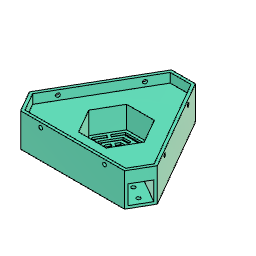
lower_connector (Autodesk Fusion 360 design; units mm, degrees)
Autodesk Fusion 360 part; units mm, degrees
sketch "Sketch1" plane through (0, 0, 0) normal (0, 0, 1) x (1, 0, 0)
  line L0 (-26, 0) -> (-82.282, -97.4833)
  line L1 (-69.282, -120) -> (43.282, -120)
  line L2 (56.282, -97.4833) -> (0, 0)
  line L3 (49.782, -108.7417) -> (-54.141, -48.7417) construction
  line L4 (0, 0) -> (-26, 0)
  line L5 (-82.282, -97.4833) -> (-69.282, -120)
  line L6 (43.282, -120) -> (56.282, -97.4833)
  line L7 (-13, 0) -> (-13, -120) construction
  line L8 (-75.782, -108.7417) -> (28.141, -48.7417) construction
  line L9 (-24.2679, -3) -> (-78.8179, -97.4833)
  line L10 (-78.8179, -97.4833) -> (-67.55, -117)
  line L11 (-67.55, -117) -> (41.55, -117)
  line L12 (41.55, -117) -> (52.8179, -97.4833)
  line L13 (52.8179, -97.4833) -> (-1.7321, -3)
  line L14 (-1.7321, -3) -> (-24.2679, -3)
  line L15 (2, -98.4752) -> (-28, -98.4752)
  line L16 (-28, -98.4752) -> (-43, -72.4944)
  line L17 (-43, -72.4944) -> (-28, -46.5137)
  line L18 (-28, -46.5137) -> (2, -46.5137)
  line L19 (2, -46.5137) -> (17, -72.4944)
  line L20 (17, -72.4944) -> (2, -98.4752)
  point P0 (-13, -72.4944)
  dimension "d18" = 120
  dimension "d25" = -3
  dimension "d36" = 26
  dimension "d42" = 30
  constraint coincident L2.end L4.start
  constraint horizontal L1
  constraint midpoint L0 L3.end
  constraint coincident L3 P0
  constraint symmetric L1.end L2.start L3
  constraint coincident L3.start L6
  constraint horizontal L4
  constraint midpoint L4 L7.start
  constraint midpoint L1 L7.end
  constraint midpoint L5 L8.start
  constraint midpoint L2 L8.end
  constraint coincident P0 L8
  constraint coincident P0 L7
  constraint perpendicular L4 L7
  constraint perpendicular L5 L8
  constraint symmetric L0 L1 L8
  constraint symmetric L0 L2 L7
  constraint equal L1 L2
  constraint horizontal L15
  constraint perpendicular L8 L16
  constraint parallel L15 L18
  constraint perpendicular L3 L20
  constraint perpendicular L8 L19
  constraint perpendicular L3 L17
  constraint symmetric L7 L16 L20
  constraint symmetric L7 L17 L19
  constraint symmetric L3 L16 L18
  constraint symmetric L3 L15 L19
  constraint equal L15 L16
  measures "d18" distance of L2.end L1
  measures "d36" distance of L1.end L2.start
  measures "d42" distance of L15.start L15.end
extrude "Extrude7" add sketch "Sketch1" along normal blind 2 contours L15 L16 L17 L18 L19 L20
extrude "Extrude4" add sketch "Sketch1" along normal blind 26 contours L0 L1 L2 L4 L5 L6 | L9 L10 L11 L12 L13 L14
sketch "Sketch2" plane through (84.423, -48.7417, 0) normal (0.866025, -0.5, 0) x (0.5, 0.866025, 0)
  line L0 (-82.282, 0) -> (-56.282, 0)
  line L1 (-56.282, 0) -> (-56.282, 26)
  line L2 (-56.282, 26) -> (-82.282, 26)
  line L3 (-82.282, 26) -> (-82.282, 0)
  line L4 (-82.282, 0) -> (-56.282, 26) construction
  line L5 (-56.282, 0) -> (-82.282, 26) construction
  line L6 (-79.482, 2.8) -> (-59.082, 2.8)
  line L7 (-59.082, 2.8) -> (-59.082, 23.2)
  line L8 (-59.082, 23.2) -> (-79.482, 23.2)
  line L9 (-79.482, 23.2) -> (-79.482, 2.8)
  dimension "d79" = 20.4
  constraint coincident L0.start L3.end
  constraint coincident L1.end L2.start
  constraint coincident L0.end L1.start
  constraint coincident L2.end L3.start
  constraint horizontal L6
  constraint vertical L7
  constraint horizontal L8
  constraint vertical L9
  constraint coincident L4 L7.end
  constraint coincident L4 L6.start
  constraint coincident L5 L8.end
  measures "d79" distance of L7.end L8.end
extrude "Extrude5" cut sketch "Sketch2" against normal blind 30 contours L6 L7 L8 L9
sketch "Sketch8" plane through (0, 0, 0) normal (0, 1, 0) x (-1, 0, 0)
  line L0 (0, 0) -> (26, 0)
  line L1 (26, 0) -> (26, 26)
  line L2 (26, 26) -> (0, 26)
  line L3 (0, 26) -> (0, 0)
  line L4 (0, 0) -> (26, 26) construction
  line L5 (0, 26) -> (26, 0) construction
  line L6 (2.8, 2.8) -> (23.2, 2.8)
  line L7 (23.2, 2.8) -> (23.2, 23.2)
  line L8 (23.2, 23.2) -> (2.8, 23.2)
  line L9 (2.8, 23.2) -> (2.8, 2.8)
  dimension "d62" = 20.4
  constraint coincident L0.start L3.end
  constraint coincident L1.end L2.start
  constraint coincident L2.end L3.start
  constraint coincident L0.end L1.start
  constraint horizontal L6
  constraint vertical L7
  constraint horizontal L8
  constraint vertical L9
  constraint coincident L4 L7.end
  constraint coincident L4 L6.start
  constraint coincident L5 L8.end
  measures "d62" distance of L7.end L8.end
extrude "Extrude9" cut sketch "Sketch8" against normal blind 30 contours L6 L7 L8 L9
sketch "Sketch9" plane through (-103.923, -60, 0) normal (-0.866025, -0.5, 0) x (0.5, -0.866025, 0)
  line L0 (43.282, 0) -> (69.282, 0)
  line L1 (69.282, 0) -> (69.282, 26)
  line L2 (69.282, 26) -> (43.282, 26)
  line L3 (43.282, 26) -> (43.282, 0)
  line L4 (43.282, 0) -> (69.282, 26) construction
  line L5 (43.282, 26) -> (69.282, 0) construction
  line L6 (46.082, 2.8) -> (66.482, 2.8)
  line L7 (66.482, 2.8) -> (66.482, 23.2)
  line L8 (66.482, 23.2) -> (46.082, 23.2)
  line L9 (46.082, 23.2) -> (46.082, 2.8)
  dimension "d65" = 20.4
  constraint coincident L0.start L3.end
  constraint coincident L1.end L2.start
  constraint coincident L2.end L3.start
  constraint coincident L0.end L1.start
  constraint horizontal L6
  constraint vertical L7
  constraint horizontal L8
  constraint vertical L9
  constraint coincident L4 L7.end
  constraint coincident L4 L6.start
  constraint coincident L5 L8.end
  measures "d65" distance of L7.end L8.end
extrude "Extrude10" cut sketch "Sketch9" against normal blind 30 contours L6 L7 L8 L9
sketch "Sketch7" plane through (0, 0, 2) normal (0, 0, 1) x (-1, 0, 0)
  line L0 (14.5, 80.4752, 24) -> (14.5, 83.4752, 24)
  line L1 (17.6077, 80.4752, 24) -> (14.5, 80.4752, 24)
  line L2 (24.3577, 80.7839, 24) -> (26.9558, 82.2839, 24)
  line L3 (18.7513, 72.4944, 24) -> (18.0635, 73.6858, 24)
  line L4 (25.6795, 72.4944, 24) -> (19.3397, 83.4752, 24)
  line L5 (22.2154, 72.4944, 24) -> (20.6615, 75.1858, 24)
  line L6 (19.1615, 77.7839, 24) -> (17.6077, 80.4752, 24)
  line L7 (24.3577, 80.7839, 24) -> (21.0718, 86.4752, 24)
  line L8 (20.6615, 75.1858, 24) -> (19.1615, 77.7839, 24)
  line L9 (19.3397, 83.4752, 24) -> (14.5, 83.4752, 24)
  line L10 (18.0635, 73.6858, 24) -> (20.6615, 75.1858, 24)
  line L11 (25.8577, 78.1858, 24) -> (28.4558, 79.6858, 24)
  line L12 (16.5635, 76.2839, 24) -> (15.8756, 77.4752, 24)
  line L13 (18.0635, 73.6858, 24) -> (16.5635, 76.2839, 24)
  line L14 (15.8756, 77.4752, 24) -> (10.1244, 77.4752, 24)
  line L15 (16.5635, 76.2839, 24) -> (19.1615, 77.7839, 24)
  line L16 (26.2679, 95.4752, 24) -> (14.5, 95.4752, 24)
  line L17 (24.5359, 92.4752, 24) -> (14.5, 92.4752, 24)
  line L18 (29.1436, 72.4944, 24) -> (25.8577, 78.1858, 24)
  line L19 (6.6603, 61.5137, 24) -> (19.3397, 61.5137, 24)
  line L20 (26.9558, 82.2839, 24) -> (22.8038, 89.4752, 24)
  line L21 (14.5, 58.5137, 24) -> (21.0718, 58.5137, 24)
  line L22 (14.5, 55.5137, 24) -> (22.8038, 55.5137, 24)
  line L23 (11.5, 64.5137, 24) -> (14.5, 64.5137, 24)
  line L24 (14.5, 92.4752, 24) -> (14.5, 95.4752, 24)
  line L25 (19.3397, 61.5137, 24) -> (21.7596, 65.705, 24)
  line L26 (17.6077, 64.5137, 24) -> (19.1615, 67.205, 24)
  line L27 (32.6077, 72.4944, 24) -> (28.4558, 79.6858, 24)
  line L28 (34.75, 58.205, 24) -> (-10.25, 84.1858, 24) construction
  line L29 (4.2404, 65.705, 24) -> (2.7404, 68.3031, 24)
  line L30 (3.1962, 55.5137, 24) -> (11.5, 55.5137, 24)
  line L31 (10.1244, 67.5137, 24) -> (11.5, 67.5137, 24)
  line L32 (5.3385, 69.8031, 24) -> (2.7404, 68.3031, 24)
  line L33 (3.7846, 72.4944, 24) -> (5.3385, 69.8031, 24)
  line L34 (7.2487, 72.4944, 24) -> (10.1244, 67.5137, 24)
  line L35 (-0.2679, 49.5137, 24) -> (26.2679, 49.5137, 24)
  line L36 (0.3205, 72.4944, 24) -> (2.7404, 68.3031, 24)
  line L37 (6.8385, 67.205, 24) -> (5.3385, 69.8031, 24)
  line L38 (-13.5359, 72.4944, 24) -> (-7.6519, 62.3031, 24)
  line L39 (-2, 46.5137, 24) -> (28, 46.5137, 24)
  line L40 (-2, 98.4752, 24) -> (-17, 72.4944, 24)
  line L41 (11.5, 98.4752, 24) -> (11.5, 46.5137, 24) construction
  line L42 (-6.6077, 72.4944, 24) -> (3.1962, 55.5137, 24)
  line L43 (-17, 72.4944, 24) -> (-2, 46.5137, 24)
  line L44 (11.5, 67.5137, 24) -> (11.5, 64.5137, 24)
  line L45 (8.3923, 64.5137, 24) -> (11.5, 64.5137, 24)
  line L46 (34.75, 86.7839, 24) -> (-10.25, 60.8031, 24) construction
  line L47 (11.5, 58.5137, 24) -> (11.5, 55.5137, 24)
  line L48 (4.2404, 65.705, 24) -> (6.6603, 61.5137, 24)
  line L49 (6.8385, 67.205, 24) -> (4.2404, 65.705, 24)
  line L50 (6.8385, 67.205, 24) -> (8.3923, 64.5137, 24)
  line L51 (-3.5538, 61.205, 24) -> (1.4641, 52.5137, 24)
  line L52 (-9.5, 59.5041, 24) -> (35.5, 85.4848, 24) construction
  line L53 (4.9282, 58.5137, 24) -> (11.5, 58.5137, 24)
  line L54 (-10.0718, 72.4944, 24) -> (-5.0538, 63.8031, 24)
  line L55 (36.25, 84.1858, 24) -> (-8.75, 58.205, 24) construction
  line L56 (23.2596, 68.3031, 24) -> (25.6795, 72.4944, 24)
  line L57 (15.8756, 67.5137, 24) -> (18.7513, 72.4944, 24)
  line L58 (26.2679, 49.5137, 24) -> (32.1519, 59.705, 24)
  line L59 (31.0538, 63.8031, 24) -> (36.0718, 72.4944, 24)
  line L60 (22.8038, 55.5137, 24) -> (32.6077, 72.4944, 24)
  line L61 (19.1615, 67.205, 24) -> (21.7596, 65.705, 24)
  line L62 (36.0718, 72.4944, 24) -> (24.5359, 92.4752, 24)
  line L63 (14.5, 64.5137, 24) -> (17.6077, 64.5137, 24)
  line L64 (43, 72.4944, 24) -> (28, 98.4752, 24)
  line L65 (39.5359, 72.4944, 24) -> (26.2679, 95.4752, 24)
  line L66 (29.5538, 61.205, 24) -> (32.1519, 59.705, 24)
  line L67 (19.1615, 67.205, 24) -> (20.6615, 69.8031, 24)
  line L68 (21.7596, 65.705, 24) -> (23.2596, 68.3031, 24)
  line L69 (28, 46.5137, 24) -> (43, 72.4944, 24)
  line L70 (14.5, 67.5137, 24) -> (15.8756, 67.5137, 24)
  line L71 (11.5, 67.5137, 24) -> (14.5, 67.5137, 24)
  line L72 (14.5, 64.5137, 24) -> (14.5, 67.5137, 24)
  line L73 (23.2596, 68.3031, 24) -> (20.6615, 69.8031, 24)
  line L74 (14.5, 55.5137, 24) -> (14.5, 58.5137, 24)
  line L75 (14.5, 46.5137, 24) -> (14.5, 98.4752, 24) construction
  line L76 (21.0718, 58.5137, 24) -> (29.1436, 72.4944, 24)
  line L77 (24.5359, 52.5137, 24) -> (29.5538, 61.205, 24)
  line L78 (20.6615, 69.8031, 24) -> (22.2154, 72.4944, 24)
  line L79 (5.3385, 75.1858, 24) -> (6.8385, 77.7839, 24)
  line L80 (13, 98.4752, 24) -> (13, 46.5137, 24) construction
  line L81 (33.6519, 62.3031, 24) -> (39.5359, 72.4944, 24)
  line L82 (33.6519, 62.3031, 24) -> (31.0538, 63.8031, 24)
  line L83 (1.4641, 52.5137, 24) -> (24.5359, 52.5137, 24)
  line L84 (-3.1436, 72.4944, 24) -> (4.9282, 58.5137, 24)
  line L85 (36.25, 60.8031, 24) -> (-8.75, 86.7839, 24) construction
  line L86 (35.5, 59.5041, 24) -> (-9.5, 85.4848, 24) construction
  line L87 (1.4641, 92.4752, 24) -> (-10.0718, 72.4944, 24)
  line L88 (-0.2679, 95.4752, 24) -> (-13.5359, 72.4944, 24)
  line L89 (-3.5538, 61.205, 24) -> (-6.1519, 59.705, 24)
  line L90 (22.8038, 89.4752, 24) -> (3.1962, 89.4752, 24)
  line L91 (11.5, 83.4752, 24) -> (6.6603, 83.4752, 24)
  line L92 (8.3923, 80.4752, 24) -> (6.8385, 77.7839, 24)
  line L93 (5.3385, 75.1858, 24) -> (3.7846, 72.4944, 24)
  line L94 (28, 98.4752, 24) -> (-2, 98.4752, 24)
  line L95 (3.1962, 89.4752, 24) -> (-0.9558, 82.2839, 24)
  line L96 (11.5, 92.4752, 24) -> (1.4641, 92.4752, 24)
  line L97 (-5.0538, 63.8031, 24) -> (-7.6519, 62.3031, 24)
  line L98 (11.5, 83.4752, 24) -> (11.5, 80.4752, 24)
  line L99 (21.0718, 86.4752, 24) -> (4.9282, 86.4752, 24)
  line L100 (-6.1519, 59.705, 24) -> (-0.2679, 49.5137, 24)
  line L101 (4.9282, 86.4752, 24) -> (1.6423, 80.7839, 24)
  line L102 (-2.4558, 79.6858, 24) -> (-6.6077, 72.4944, 24)
  line L103 (-2.4558, 79.6858, 24) -> (0.1423, 78.1858, 24)
  line L104 (11.5, 95.4752, 24) -> (-0.2679, 95.4752, 24)
  line L105 (2.7404, 76.6858, 24) -> (0.3205, 72.4944, 24)
  line L106 (4.2404, 79.2839, 24) -> (2.7404, 76.6858, 24)
  line L107 (7.9365, 73.6858, 24) -> (7.2487, 72.4944, 24)
  line L108 (11.5, 95.4752, 24) -> (11.5, 92.4752, 24)
  line L109 (10.1244, 77.4752, 24) -> (9.4365, 76.2839, 24)
  line L110 (1.6423, 80.7839, 24) -> (-0.9558, 82.2839, 24)
  line L111 (11.5, 80.4752, 24) -> (8.3923, 80.4752, 24)
  line L112 (9.4365, 76.2839, 24) -> (6.8385, 77.7839, 24)
  line L113 (7.9365, 73.6858, 24) -> (5.3385, 75.1858, 24)
  line L114 (7.9365, 73.6858, 24) -> (9.4365, 76.2839, 24)
  line L115 (0.1423, 78.1858, 24) -> (-3.1436, 72.4944, 24)
  line L116 (6.6603, 83.4752, 24) -> (4.2404, 79.2839, 24)
  dimension "d80" = 3
  dimension "d81" = 3
  dimension "d82" = 3
  dimension "d83" = 3
  dimension "d84" = 3
  dimension "d85" = 3
  dimension "d86" = 6
  dimension "d87" = 6
  dimension "d88" = 6
  dimension "d89" = 6
  dimension "d90" = 6
  dimension "d91" = 6
  dimension "d92" = 9
  dimension "d93" = 9
  dimension "d94" = 9
  dimension "d95" = 9
  dimension "d96" = 9
  dimension "d97" = 9
  dimension "d98" = 12
  dimension "d99" = 12
  dimension "d100" = 12
  dimension "d101" = 12
  dimension "d102" = 12
  dimension "d103" = 12
  dimension "d104" = 18
  dimension "d105" = 18
  dimension "d106" = 18
  dimension "d107" = 18
  dimension "d108" = 18
  dimension "d109" = 18
  dimension "d110" = 15
  dimension "d111" = 15
  dimension "d112" = 15
  dimension "d113" = 15
  dimension "d114" = 15
  dimension "d115" = 15
  dimension "d116" = 3
  dimension "d117" = 3
  dimension "d118" = 3
  dimension "d119" = 21
  dimension "d120" = 21
  dimension "d121" = 21
  dimension "d122" = 21
  dimension "d123" = 21
  dimension "d124" = 21
extrude "Extrude8" cut sketch "Sketch7" against normal blind 65 contours L0 L1 L4 L5 L6 L8 L9 L56 L73 L78 | L3 L12 L13 L14 L31 L34 L57 L70 L71 L107 L109 L114 | L19 L23 L25 L26 L45 L48 L49 L50 L61 L63 | L32 L33 L36 L79 L91 L92 L93 L98 L105 L106 L111 L116 | L2 L7 L20 L90 L95 L99 L101 L110 | L11 L18 L21 L22 L27 L60 L74 L76 | L16 L17 L24 L59 L62 L65 L81 L82 | L30 L42 L47 L53 L84 L102 L103 L115 | L35 L51 L58 L66 L77 L83 L89 L100 | L38 L54 L87 L88 L96 L97 L104 L108 in plane through (0, 0, 26) normal (0, 0, 1)
sketch "Sketch13" plane through (0, 0, 0) normal (0, 0, -1) x (1, 0, 0)
  line L0 (-6.6603, 83.4752) -> (-0.3205, 72.4944)
  line L1 (-0.3205, 72.4944) -> (-2.7404, 68.3031)
  line L2 (-2.7404, 68.3031) -> (-5.3385, 69.8031)
  line L3 (-5.3385, 69.8031) -> (-3.7846, 72.4944)
  line L4 (-3.7846, 72.4944) -> (-8.3923, 80.4752)
  line L5 (-8.3923, 80.4752) -> (-11.5, 80.4752)
  line L6 (-11.5, 80.4752) -> (-11.5, 83.4752)
  line L7 (-11.5, 83.4752) -> (-6.6603, 83.4752)
  line L8 (6.6077, 72.4944) -> (-3.1962, 55.5137)
  line L9 (-3.1962, 55.5137) -> (-11.5, 55.5137)
  line L10 (-11.5, 55.5137) -> (-11.5, 58.5137)
  line L11 (-11.5, 58.5137) -> (-4.9282, 58.5137)
  line L12 (-4.9282, 58.5137) -> (3.1436, 72.4944)
  line L13 (3.1436, 72.4944) -> (-0.1423, 78.1858)
  line L14 (-0.1423, 78.1858) -> (2.4558, 79.6858)
  line L15 (2.4558, 79.6858) -> (6.6077, 72.4944)
  line L16 (-26.2679, 95.4752) -> (-14.5, 95.4752)
  line L17 (-14.5, 95.4752) -> (-14.5, 92.4752)
  line L18 (-14.5, 92.4752) -> (-24.5359, 92.4752)
  line L19 (-24.5359, 92.4752) -> (-36.0718, 72.4944)
  line L20 (-36.0718, 72.4944) -> (-31.0538, 63.8031)
  line L21 (-31.0538, 63.8031) -> (-33.6519, 62.3031)
  line L22 (-33.6519, 62.3031) -> (-39.5359, 72.4944)
  line L23 (-39.5359, 72.4944) -> (-26.2679, 95.4752)
  line L24 (6.1519, 59.705) -> (0.2679, 49.5137)
  line L25 (0.2679, 49.5137) -> (-26.2679, 49.5137)
  line L26 (-26.2679, 49.5137) -> (-32.1519, 59.705)
  line L27 (-32.1519, 59.705) -> (-29.5538, 61.205)
  line L28 (-29.5538, 61.205) -> (-24.5359, 52.5137)
  line L29 (-24.5359, 52.5137) -> (-1.4641, 52.5137)
  line L30 (-1.4641, 52.5137) -> (3.5538, 61.205)
  line L31 (3.5538, 61.205) -> (6.1519, 59.705)
  line L32 (-4.2404, 65.705) -> (-6.6603, 61.5137)
  line L33 (-6.6603, 61.5137) -> (-19.3397, 61.5137)
  line L34 (-19.3397, 61.5137) -> (-21.7596, 65.705)
  line L35 (-21.7596, 65.705) -> (-19.1615, 67.205)
  line L36 (-19.1615, 67.205) -> (-17.6077, 64.5137)
  line L37 (-17.6077, 64.5137) -> (-8.3923, 64.5137)
  line L38 (-8.3923, 64.5137) -> (-6.8385, 67.205)
  line L39 (-6.8385, 67.205) -> (-4.2404, 65.705)
  line L40 (-25.6795, 72.4944) -> (-19.3397, 83.4752)
  line L41 (-19.3397, 83.4752) -> (-14.5, 83.4752)
  line L42 (-14.5, 83.4752) -> (-14.5, 80.4752)
  line L43 (-14.5, 80.4752) -> (-17.6077, 80.4752)
  line L44 (-17.6077, 80.4752) -> (-22.2154, 72.4944)
  line L45 (-22.2154, 72.4944) -> (-20.6615, 69.8031)
  line L46 (-20.6615, 69.8031) -> (-23.2596, 68.3031)
  line L47 (-23.2596, 68.3031) -> (-25.6795, 72.4944)
  line L48 (-26.9558, 82.2839) -> (-22.8038, 89.4752)
  line L49 (-22.8038, 89.4752) -> (-3.1962, 89.4752)
  line L50 (-3.1962, 89.4752) -> (0.9558, 82.2839)
  line L51 (0.9558, 82.2839) -> (-1.6423, 80.7839)
  line L52 (-1.6423, 80.7839) -> (-4.9282, 86.4752)
  line L53 (-4.9282, 86.4752) -> (-21.0718, 86.4752)
  line L54 (-21.0718, 86.4752) -> (-24.3577, 80.7839)
  line L55 (-24.3577, 80.7839) -> (-26.9558, 82.2839)
  line L56 (13.5359, 72.4944) -> (7.6519, 62.3031)
  line L57 (7.6519, 62.3031) -> (5.0538, 63.8031)
  line L58 (5.0538, 63.8031) -> (10.0718, 72.4944)
  line L59 (10.0718, 72.4944) -> (-1.4641, 92.4752)
  line L60 (-1.4641, 92.4752) -> (-11.5, 92.4752)
  line L61 (-11.5, 92.4752) -> (-11.5, 95.4752)
  line L62 (-11.5, 95.4752) -> (0.2679, 95.4752)
  line L63 (0.2679, 95.4752) -> (13.5359, 72.4944)
  line L64 (-22.8038, 55.5137) -> (-32.6077, 72.4944)
  line L65 (-32.6077, 72.4944) -> (-28.4558, 79.6858)
  line L66 (-28.4558, 79.6858) -> (-25.8577, 78.1858)
  line L67 (-25.8577, 78.1858) -> (-29.1436, 72.4944)
  line L68 (-29.1436, 72.4944) -> (-21.0718, 58.5137)
  line L69 (-21.0718, 58.5137) -> (-14.5, 58.5137)
  line L70 (-14.5, 58.5137) -> (-14.5, 55.5137)
  line L71 (-14.5, 55.5137) -> (-22.8038, 55.5137)
  line L72 (-10.1244, 67.5137) -> (-15.8756, 67.5137)
  line L73 (-15.8756, 67.5137) -> (-18.7513, 72.4944)
  line L74 (-18.7513, 72.4944) -> (-15.8756, 77.4752)
  line L75 (-15.8756, 77.4752) -> (-10.1244, 77.4752)
  line L76 (-10.1244, 77.4752) -> (-7.2487, 72.4944)
  line L77 (-7.2487, 72.4944) -> (-10.1244, 67.5137)
  line L78 (56.282, 97.4833) -> (43.282, 120)
  line L79 (43.282, 120) -> (-69.282, 120)
  line L80 (-69.282, 120) -> (-82.282, 97.4833)
  line L81 (-82.282, 97.4833) -> (-26, 0)
  line L82 (-26, 0) -> (0, 0)
  line L83 (0, 0) -> (56.282, 97.4833)
  line L84 (-13, 0) -> (-13, 72.4944) construction
  line L85 (-13, 72.4944) -> (49.782, 108.7417) construction
  line L86 (-13, 72.4944) -> (-75.782, 108.7417) construction
  circle A0 centre (-13, 7.5) radius 2
  circle A1 centre (-13, 22.5) radius 2
  circle A2 centre (43.2868, 104.9917) radius 2
  circle A3 centre (30.2965, 97.4917) radius 2
  circle A4 centre (-69.2868, 104.9917) radius 2
  circle A5 centre (-56.2965, 97.4917) radius 2
  dimension "d136" = 4
  dimension "d137" = 7.5
  dimension "d138" = 15
  dimension "d139" = 7.5
  dimension "d140" = 15
  dimension "d141" = 7.5
  dimension "d142" = 15
  constraint midpoint L82 L84.start
  constraint perpendicular L82 L84
  constraint midpoint L78 L85.end
  constraint midpoint L80 L86.end
  constraint perpendicular L80 L86
  constraint coincident L84 A0.centre
  constraint coincident L84 A1.centre
  constraint coincident L85 A2.centre
  constraint coincident L85 A3.centre
  constraint coincident L86 A4.centre
  constraint coincident L86 A5.centre
  constraint equal A0 A1
  constraint equal A1 A5
  constraint equal A4 A5
  constraint equal A3 A4
  constraint equal A2 A3
  measures "d136" diameter of A2
  measures "d137" distance of L78 A2.centre
  measures "d138" distance of A2.centre A3.centre
  measures "d139" distance of L82 A0.centre
  measures "d140" distance of A0.centre A1.centre
  measures "d141" distance of L80 A4.centre
  measures "d142" distance of A4.centre A5.centre
extrude "Extrude14" cut sketch "Sketch13" against normal blind 10 contours A0 | A1 | A2 | A3 | A4 | A5
extrude "Extrude16" add sketch "Sketch1" along normal blind 10 from surface at 26 contours L0 L1 L2 L4 L5 L6
sketch "Sketch17" plane through (-16.9019, 9.7583, 0) normal (0.866025, -0.5, 0) x (0.5, 0.866025, 0)
  line L0 (-123.832, 26) -> (-14.7321, 26)
  line L1 (-14.7321, 26) -> (-14.7321, 36)
  line L2 (-14.7321, 36) -> (-123.832, 36)
  line L3 (-123.832, 36) -> (-123.832, 26)
  line L4 (-123.832, 31) -> (-14.7321, 31) construction
  line L5 (-69.282, 26) -> (-69.282, 36) construction
  circle A0 centre (-103.832, 31) radius 2
  circle A1 centre (-34.7321, 31) radius 2
  dimension "d154" = 20
  dimension "d155" = 4
  constraint midpoint L3 L4.start
  constraint midpoint L1 L4.end
  constraint midpoint L0 L5.start
  constraint midpoint L2 L5.end
  constraint coincident L4 A0.centre
  constraint coincident L4 A1.centre
  constraint equal A0 A1
  constraint symmetric L5 A0 A1
  measures "d154" distance of L4.start A0.centre
  measures "d155" diameter of A0
sketch "Sketch19" plane through (-2.5981, -1.5, 0) normal (-0.866025, -0.5, 0) x (0.5, -0.866025, 0)
  line L0 (1.7321, 26) -> (110.832, 26)
  line L1 (110.832, 26) -> (110.832, 36)
  line L2 (110.832, 36) -> (1.7321, 36)
  line L3 (1.7321, 36) -> (1.7321, 26)
  line L4 (1.7321, 31) -> (110.832, 31) construction
  line L5 (56.282, 26) -> (56.282, 36) construction
  circle A0 centre (90.832, 31) radius 2
  circle A1 centre (21.7321, 31) radius 2
  dimension "d156" = 20
  dimension "d157" = 4
  constraint coincident A1.centre L4
  constraint coincident A0.centre L4
  constraint equal A0 A1
  constraint symmetric L5 A0 A1
  constraint coincident L3 L4.start
  constraint coincident L2 L5.end
  constraint coincident L0 L5.start
  constraint coincident L1 L4.end
  constraint midpoint L1 L4.end
  constraint midpoint L2 L5.end
  constraint midpoint L0 L5.start
  measures "d156" distance of A1.centre L4.start
  measures "d157" diameter of A1
sketch "Sketch20" plane through (0, -117, 0) normal (0, 1, 0) x (-1, 0, 0)
  line L0 (-41.55, 26) -> (67.55, 26)
  line L1 (67.55, 26) -> (67.55, 36)
  line L2 (67.55, 36) -> (-41.55, 36)
  line L3 (-41.55, 36) -> (-41.55, 26)
  line L4 (-41.55, 31) -> (67.55, 31) construction
  line L5 (13, 26) -> (13, 36) construction
  circle A0 centre (47.55, 31) radius 2
  circle A1 centre (-21.55, 31) radius 2
  dimension "d158" = 20
  dimension "d159" = 4
  constraint coincident A1.centre L4
  constraint coincident A0.centre L4
  constraint equal A0 A1
  constraint symmetric L5 A0 A1
  constraint midpoint L3 L4.start
  constraint midpoint L0 L5.start
  constraint midpoint L2 L5.end
  constraint midpoint L1 L4.end
  measures "d158" distance of A1.centre L4.start
  measures "d159" diameter of A1
extrude "Extrude17" cut sketch "Sketch20" against normal blind 5 contours A0 | A1
extrude "Extrude18" cut sketch "Sketch19" against normal blind 5 contours A0 | A1
extrude "Extrude19" cut sketch "Sketch17" against normal blind 5 contours A0 | A1
equation "gap = 0.2 mm"
equation "d62 = 20 mm + 2 * gap"
equation "d65 = 20 mm + 2 * gap"
equation "d79 = 20 mm + 2 * gap"
